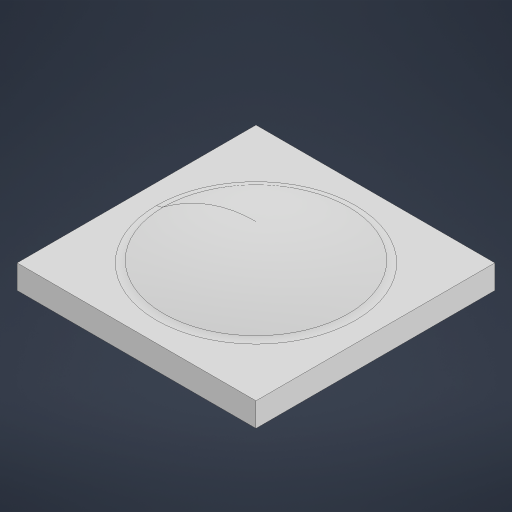
# Autodesk Inventor part: Surface1
Saved by Autodesk Inventor 2024.3 (Build 283343000, 343)
## iProperties
Created: 2024-10-21
Part Number: Surface1
Material: Generic
Document SubType Name: Modeling
Designer: fablabadmin
Density: 1 g/cm^3
Appearance: Default
Author: fablabadmin
Autodesk Inventor part; units mm, degrees
ref_plane "YZ Plane" through (0, 0, 0) normal (1, 0, 0) x (0, 1, 0)
ref_plane "XZ Plane" through (0, 0, 0) normal (0, 1, 0) x (-1, 0, 0)
ref_plane "XY Plane" through (0, 0, 0) normal (0, 0, 1) x (1, 0, 0)
sketch "Sketch1" plane through (0, 0, 0) normal (0, 1, 0) x (-1, 0, 0)
  line L0 (-50, 50) -> (50, 50)
  line L1 (50, 50) -> (50, -50)
  line L2 (50, -50) -> (-50, -50)
  line L3 (-50, -50) -> (-50, 50)
  line L4 (-50, 50) -> (50, -50) construction
  line L5 (50, 50) -> (-50, -50) construction
  point P0 (0, 0)
  dimension "d0" = 100
  constraints: 12 end point, 2 midpoint, 2 parallel, 2 perpendicular, 1 horizontal
  measures "d0" distance of L1.end L2.end
sketch "Sketch2" plane through (0, 0, 0) normal (0, 0, 1) x (1, 0, 0)
  line L0 (0, -6.18) -> (0, 36.03) projected
  line L1 (50, 0) -> (-50, 0) projected
  line L2 (-40, 0) -> (0, 30) construction
  line L3 (0, 30) -> (40, 0) construction
  spline S0 degree 2 poles (-40, 0) (0, 30) (40, 0) knots 1 1 1 2 2 2
  point P0 (0, 0)
  point P1 (0, 0)
  point P2 (0, 15)
  dimension "d1" = 30
  dimension "d2" = 10
  constraints: 4 point on line, 1 midpoint, 1 symmetric about line, 4 other
  measures "d1" distance of point (0, 0) L2.end
  measures "d2" distance of L2.start L1.end
extrude "Extrusion1" add sketch "Sketch1" against normal blind 10
revolve "Revolution2" add sketch "Sketch2" angle 360 about axis through (0, -10, 0) along (0, 1, 0) picked at (-23.2026, 2.2606) contours L1 S0 L0
fillet "Fillet1" radius 5 1 edges at (40, 0, 0)
body "Solid1"
